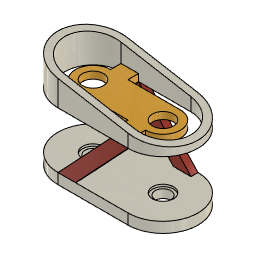
Exercise-23 v1 (Autodesk Fusion 360 design; units mm, degrees)
Autodesk Fusion 360 part; units mm, degrees
sketch "Sketch1" plane through (0, 0, 0) normal (0, 0, 1) x (1, 0, 0)
  line L0 (0, 50) -> (-100, 50)
  arc A0 (-100, 50) -> (-100, -50) centre (-100, 0) ccw
  line L1 (-100, -50) -> (0, -50)
  arc A1 (0, -50) -> (0, 50) centre (0, 0) ccw
  line L2 (0, 0) -> (-100, 0) construction
  arc A2 (0, -40) -> (0, 40) centre (0, 0) ccw
  line L3 (0, 40) -> (-100, 40)
  arc A3 (-100, 40) -> (-100, -40) centre (-100, 0) ccw
  line L4 (-100, -40) -> (0, -40)
  line L5 (-100, -25) -> (0, -25)
  arc A4 (0, -25) -> (0, 25) centre (0, 0) ccw
  line L6 (0, 25) -> (-100, 25)
  arc A5 (-100, 25) -> (-100, -25) centre (-100, 0) ccw
  circle A6 centre (0, 0) radius 11.25
  circle A7 centre (0, 0) radius 15
  circle A8 centre (-100, 0) radius 11.25
  circle A9 centre (-100, 0) radius 15
  line L7 (-100, 25) -> (-75, 25)
  line L8 (-75, 25) -> (-75, 40)
  line L9 (-75, 40) -> (-100, 40)
  line L10 (-100, 40) -> (-100, 25)
  line L11 (0, -25) -> (-25, -25)
  line L12 (-25, -25) -> (-25, -40)
  line L13 (-25, -40) -> (0, -40)
  line L14 (0, -40) -> (0, -25)
  dimension "d1" = 100
  dimension "d2" = 100
  dimension "d3" = -10
  dimension "d4" = -25
  dimension "d5" = 22.5
  dimension "d6" = 30
  dimension "d7" = 22.5
  dimension "d8" = 30
  dimension "d9" = 25
  dimension "d10" = 15
  dimension "d11" = 25
  dimension "d12" = 15
  constraint tangent L0 A0
  constraint tangent A0 L1
  constraint parallel L0 L1
  constraint tangent L1 A1
  constraint tangent L0 A1
  constraint horizontal L2
  constraint coincident A1.centre L2.start
  constraint concentric A1 A6
  constraint concentric A1 A7
  constraint concentric A0 A8
  constraint concentric A8 A9
  constraint horizontal L7
  constraint vertical L8
  constraint horizontal L9
  constraint vertical L10
  constraint horizontal L11
  constraint vertical L12
  constraint horizontal L13
  constraint vertical L14
  measures "d1" distance of A1.centre A0.centre
  measures "d2" diameter of A0
  measures "d5" diameter of A6
  measures "d6" diameter of A7
  measures "d7" diameter of A8
  measures "d8" diameter of A9
  measures "d9" distance of L6.end L7.end
  measures "d10" distance of L6.end L3.end
  measures "d11" distance of L5.end L11.end
  measures "d12" distance of L5.end A2.start
extrude "Extrude1" add sketch "Sketch1" against normal blind 15 contours L0 A0 L1 A1 | A2 L3 A4 L6 L8 L14 | L4 L5 L11 L12 L13 L14 | A3 L4 L5 A5 L10 L12 | L5 A4 L6 A5 L7 L11 | L3 L6 L7 L8 L9 L10 makes body 1
extrude "Extrude2" add sketch "Sketch1" along normal blind 10 from surface at 80 separate body contours L4 L5 L11 L12 L13 L14 | L5 A4 L6 A5 L7 L11 | L3 L6 L7 L8 L9 L10 makes body 2
extrude "Extrude3" add sketch "Sketch1" along normal blind 50 from surface at 80 separate body contours L0 A0 L1 A1 makes body 3
sketch "Sketch2" plane through (0, 0, 0) normal (0, 1, 0) x (1, 0, 0)
  line L0 (-25, -80) -> (0, -80)
  line L1 (-25, -90) -> (0, -90)
  line L2 (-100, -80) -> (-25, -80)
  line L3 (-100, -90) -> (-25, -90)
  line L4 (-125, -80) -> (-100, -80)
  line L5 (-125, -90) -> (-100, -90)
  line L6 (0, -80) -> (25, -80)
  line L7 (0, -90) -> (25, -90)
  line L8 (-125, -80) -> (-125, -90)
  line L9 (25, -80) -> (25, -90)
  line L10 (-100, 0) -> (-25, -80)
  line L11 (0, -80) -> (-75, 0)
  line L12 (0, 0) -> (-100, 0)
  line L13 (-50, 0) -> (-50, -15)
  line L14 (0, 0) -> (-75, -80)
  line L15 (-100, -80) -> (-25, 0)
  line L16 (-100, -80) -> (0, -80)
  line L17 (-100, -130) -> (0, -130)
  line L18 (-150, -80) -> (-100, -80)
  line L19 (-150, -130) -> (-100, -130)
  line L20 (0, -80) -> (50, -80)
  line L21 (0, -130) -> (50, -130)
  line L22 (-150, -80) -> (-150, -130)
  line L23 (50, -80) -> (50, -130)
  line L24 (-125, -90) -> (-150, -90)
  line L25 (25, -90) -> (50, -90)
  line L26 (50, -90) -> (-150, -125.2654)
  point P0 (-100, 0)
  dimension "d21" = 10
  constraint coincident P0 L10.start
  constraint coincident L0.start L2.end
  constraint coincident L0.end L6.start
  constraint parallel L10 L11
  constraint midpoint L12 L13.start
  constraint perpendicular L12 L13
  constraint symmetric P0 L13 L12.start
  constraint symmetric L0.start L13 L14.end
  constraint symmetric L0.end L13 L2.start
  constraint symmetric L11.end L13 L15.end
  constraint coincident L5.start L8.end
  constraint coincident L22 L24.end
  constraint perpendicular L22 L24
  constraint coincident L7.end L9.end
  constraint coincident L23 L25.end
  constraint perpendicular L23 L25
  constraint coincident L22 L26.end
  measures "d21" angle of L25 L26
extrude "Extrude4" cut sketch "Sketch2" along normal through all and the other way through all contours L17 L19 L21 L22 L23 L26 bodies 3
extrude "Extrude5" add sketch "Sketch2" along normal blind 10 from surface at -50 separate body contours L0 L10 L11 L14 L16 | L10 L11 L14 L15 | L10 L11 L12 L15 makes body 4
extrude "Extrude6" add sketch "Sketch2" against normal blind 10 from surface at 50 separate body contours L2 L10 L14 L15 L16 | L10 L11 L14 L15 | L11 L12 L14 L15 makes body 5
extrude "Extrude7" add sketch "Sketch1" along normal blind 12 from surface at -15 contours A7 | A9 bodies 1
